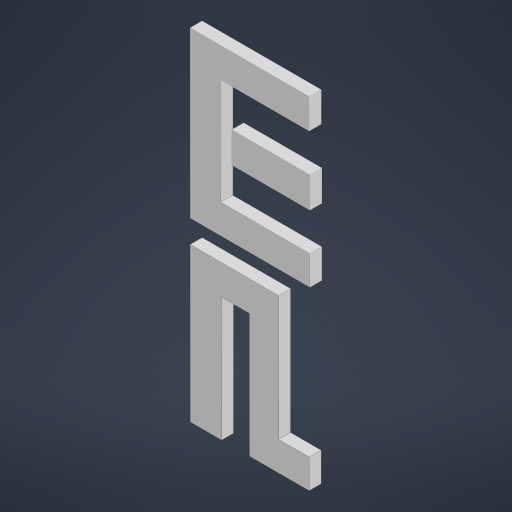
# Autodesk Inventor part: ROBOILO LOGO
Saved by Autodesk Inventor 2024 (Build 280153000, 153)
## iProperties
Created: 2024-06-09
Part Number: ROBOILO LOGO
Material: Generic
Document SubType Name: Modeling
Designer: mateu
Density: 1 g/cm^3
Appearance: Default
Author: mateu
Autodesk Inventor part; units mm, degrees
ref_plane "YZ Plane" through (0, 0, 0) normal (1, 0, 0) x (0, 1, 0)
ref_plane "XZ Plane" through (0, 0, 0) normal (0, 1, 0) x (-1, 0, 0)
ref_plane "XY Plane" through (0, 0, 0) normal (0, 0, 1) x (1, 0, 0)
sketch "Sketch1" plane through (0, 0, 0) normal (0, 0, 1) x (1, 0, 0)
  line L0 (-26.5523, -13.8097) -> (-23.4761, -13.8097) construction
  line L1 (-26.5523, -1.2089) -> (-26.5523, -13.8097) construction
  line L2 (-35.1023, -1.2089) -> (-26.5523, -1.2089) construction
  line L3 (-35.1023, -16.3589) -> (-35.1023, -1.2089) construction
  line L4 (-32.3273, -16.3589) -> (-35.1023, -16.3589) construction
  line L5 (-32.3273, -3.8452) -> (-32.3273, -16.3589) construction
  line L6 (-29.0999, -3.8452) -> (-32.3273, -3.8452) construction
  line L7 (-29.0999, -16.3589) -> (-29.0999, -3.8452) construction
  line L8 (-23.4761, -16.3589) -> (-29.0999, -16.3589) construction
  line L9 (-23.4761, -13.8097) -> (-23.4761, -16.3589) construction
  line L10 (-32.4023, 4.0411) -> (-23.4023, 4.0411) construction
  line L11 (-32.4023, 15.1366) -> (-32.4023, 4.0411) construction
  line L12 (-23.4769, 15.1366) -> (-32.4023, 15.1366) construction
  line L13 (-23.4769, 17.7661) -> (-23.4769, 15.1366) construction
  line L14 (-35.1023, 17.7661) -> (-23.4769, 17.7661) construction
  line L15 (-35.1023, 1.4911) -> (-35.1023, 17.7661) construction
  line L16 (-23.4023, 1.4911) -> (-35.1023, 1.4911) construction
  line L17 (-23.4023, 4.0411) -> (-23.4023, 1.4911) construction
  line L18 (-30.9023, 8.2411) -> (-30.9023, 10.9411) construction
  line L19 (-23.4023, 8.2411) -> (-30.9023, 8.2411) construction
  line L20 (-23.4023, 10.9411) -> (-23.4023, 8.2411) construction
  line L21 (-30.9023, 10.9411) -> (-23.4023, 10.9411) construction
  line L22 (-23.2769, 17.9661) -> (-23.2769, 14.9366)
  line L23 (-23.2769, 14.9366) -> (-32.2023, 14.9366)
  line L24 (-32.2023, 14.9366) -> (-32.2023, 4.2411)
  line L25 (-32.2023, 4.2411) -> (-23.2023, 4.2411)
  line L26 (-23.2023, 4.2411) -> (-23.2023, 1.2911)
  line L27 (-23.2023, 1.2911) -> (-35.3023, 1.2911)
  line L28 (-35.3023, 1.2911) -> (-35.3023, 17.9661)
  line L29 (-35.3023, 17.9661) -> (-23.2769, 17.9661)
  line L30 (-23.2023, 11.1411) -> (-23.2023, 8.0411)
  line L31 (-23.2023, 8.0411) -> (-31.1023, 8.0411)
  line L32 (-31.1023, 8.0411) -> (-31.1023, 11.1411)
  line L33 (-31.1023, 11.1411) -> (-23.2023, 11.1411)
  line L34 (-29.2999, -4.0452) -> (-32.1273, -4.0452)
  line L35 (-32.1273, -4.0452) -> (-32.1273, -16.5589)
  line L36 (-32.1273, -16.5589) -> (-35.3023, -16.5589)
  line L37 (-35.3023, -16.5589) -> (-35.3023, -1.0089)
  line L38 (-35.3023, -1.0089) -> (-26.3523, -1.0089)
  line L39 (-26.3523, -1.0089) -> (-26.3523, -13.6097)
  line L40 (-26.3523, -13.6097) -> (-23.2761, -13.6097)
  line L41 (-23.2761, -13.6097) -> (-23.2761, -16.5589)
  line L42 (-23.2761, -16.5589) -> (-29.2999, -16.5589)
  line L43 (-29.2999, -16.5589) -> (-29.2999, -4.0452)
  point P0 (0, 0)
  dimension "d2" = 0.2
  dimension "d3" = 0.2
  dimension "d4" = 0.2
  constraints: 44 end point, 19 other
  measures "d2" distance between parallel lines of L14 L29
  measures "d3" distance between parallel lines of L21 L33
  measures "d4" distance between parallel lines of L7 L43
extrude "Extrusion1" add sketch "Sketch1" along normal blind 1.2
body "Solid1"
